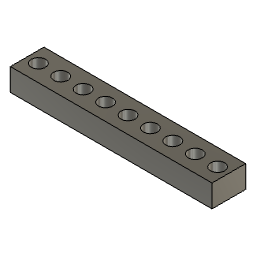
n_ext_2 v1 (Autodesk Fusion 360 design; units mm, degrees)
Autodesk Fusion 360 part; units mm, degrees
sketch "Sketch1" plane through (0, 0, 0) normal (0, 0, 1) x (1, 0, 0)
  line L0 (0, 0) -> (90, 0)
  line L1 (90, 0) -> (90, 15)
  line L2 (90, 15) -> (0, 15)
  line L3 (0, 15) -> (0, 0)
  line L4 (70, 15) -> (70, 0) construction
  line L5 (60, 15) -> (60, 0) construction
  line L6 (50, 15) -> (50, 0) construction
  line L7 (40, 15) -> (40, 0) construction
  line L8 (30, 15) -> (30, 0) construction
  line L9 (20, 15) -> (20, 0) construction
  line L10 (10, 15) -> (10, 0) construction
  line L11 (80, 15) -> (80, 0) construction
  line L12 (90, 15) -> (80, 0) construction
  line L13 (80, 15) -> (90, 0) construction
  line L14 (80, 15) -> (70, 0) construction
  line L15 (70, 15) -> (80, 0) construction
  line L16 (70, 15) -> (60, 0) construction
  line L17 (60, 15) -> (70, 0) construction
  line L18 (60, 15) -> (50, 0) construction
  line L19 (50, 15) -> (60, 0) construction
  line L20 (50, 15) -> (40, 0) construction
  line L21 (40, 15) -> (50, 0) construction
  line L22 (40, 15) -> (30, 0) construction
  line L23 (30, 15) -> (40, 0) construction
  line L24 (30, 15) -> (20, 0) construction
  line L25 (20, 15) -> (30, 0) construction
  line L26 (20, 15) -> (10, 0) construction
  line L27 (10, 15) -> (20, 0) construction
  line L28 (10, 15) -> (0, 0) construction
  line L29 (0, 15) -> (10, 0) construction
  circle A0 centre (5, 7.5) radius 3.1375
  circle A1 centre (15, 7.5) radius 3.1375
  circle A2 centre (25, 7.5) radius 3.1375
  circle A3 centre (35, 7.5) radius 3.1375
  circle A4 centre (45, 7.5) radius 3.1375
  circle A5 centre (55, 7.5) radius 3.1375
  circle A6 centre (65, 7.5) radius 3.1375
  circle A7 centre (75, 7.5) radius 3.1375
  circle A8 centre (85, 7.5) radius 3.1375
  dimension "d1" = 90
  dimension "d2" = 15
  dimension "d3" = 10
  dimension "d4" = 10
  dimension "d5" = 10
  dimension "d6" = 10
  dimension "d7" = 10
  dimension "d8" = 10
  dimension "d9" = 10
  dimension "d10" = 10
  dimension "d11" = 6.275
  dimension "d12" = 6.275
  dimension "d13" = 6.275
  dimension "d14" = 6.275
  dimension "d15" = 6.275
  dimension "d16" = 6.275
  dimension "d17" = 6.275
  dimension "d18" = 6.275
  dimension "d19" = 6.275
  constraint horizontal L0
  constraint vertical L1
  constraint horizontal L2
  constraint vertical L3
  constraint coincident L0.start L3.end
  constraint coincident L2 L4.start
  constraint coincident L0 L4.end
  constraint perpendicular L0 L4
  constraint coincident L2 L5.start
  constraint coincident L0 L5.end
  constraint perpendicular L0 L5
  constraint coincident L2 L6.start
  constraint coincident L0 L6.end
  constraint perpendicular L0 L6
  constraint coincident L2 L7.start
  constraint coincident L0 L7.end
  constraint perpendicular L0 L7
  constraint coincident L2 L8.start
  constraint coincident L0 L8.end
  constraint perpendicular L0 L8
  constraint coincident L2 L9.start
  constraint coincident L0 L9.end
  constraint perpendicular L0 L9
  constraint coincident L2 L10.start
  constraint coincident L0 L10.end
  constraint perpendicular L0 L10
  constraint coincident L2 L11.start
  constraint coincident L0 L11.end
  constraint perpendicular L0 L11
  constraint midpoint L29 A0.centre
  constraint midpoint L26 A1.centre
  constraint midpoint L24 A2.centre
  constraint midpoint L22 A3.centre
  constraint midpoint L21 A4.centre
  constraint midpoint L18 A5.centre
  constraint midpoint L16 A6.centre
  constraint midpoint L15 A7.centre
  constraint midpoint L12 A8.centre
  measures "d1" distance of L0.start L0.end
  measures "d2" distance of L0.start L2.end
  measures "d3" distance of L1 L11
  measures "d4" distance of L4 L11
  measures "d5" distance of L4 L5
  measures "d6" distance of L5 L6
  measures "d7" distance of L6 L7
  measures "d8" distance of L7 L8
  measures "d9" distance of L8 L9
  measures "d10" distance of L9 L10
  measures "d11" diameter of A0
  measures "d12" diameter of A1
  measures "d13" diameter of A2
  measures "d14" diameter of A3
  measures "d15" diameter of A4
  measures "d16" diameter of A5
  measures "d17" diameter of A6
  measures "d18" diameter of A7
  measures "d19" diameter of A8
extrude "Extrude1" add sketch "Sketch1" along normal blind 10
